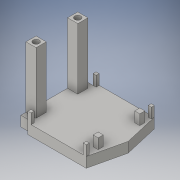
# Autodesk Inventor part: Maglev_Stand
Saved by Autodesk Inventor 2016 (Build 200138000, 138)
## iProperties
Created: 2018-01-06
Part Number: Maglev_Stand
Material: Generic
Document SubType Name: Modeling
Designer: Jorian Bruslind
Density: 1 g/cm^3
Appearance: Default
Author: Jorian Bruslind
Autodesk Inventor part; units mm, degrees
ref_plane "YZ Plane" through (0, 0, 0) normal (1, 0, 0) x (0, 1, 0)
ref_plane "XZ Plane" through (0, 0, 0) normal (0, 1, 0) x (-1, 0, 0)
ref_plane "XY Plane" through (0, 0, 0) normal (0, 0, 1) x (1, 0, 0)
sketch "Sketch1" plane through (0, 0, 0) normal (0, 1, 0) x (-1, 0, 0)
  line L0 (0, 0) -> (0, -85)
  line L1 (0, 0) -> (-60, 0)
  line L2 (-60, 0) -> (-60, -85)
  line L3 (-60, -85) -> (0, -85)
  line L4 (0, -42.5) -> (-76.2, -42.5)
  line L5 (-60, 0) -> (-66.35, 0)
  line L6 (-66.35, 0) -> (-66.35, -6.35)
  line L7 (-66.35, -6.35) -> (-60, -6.35)
  line L8 (-60, -6.35) -> (-60, 0)
  line L9 (0, 0) -> (6.35, 0)
  line L10 (6.35, 0) -> (6.35, -85)
  line L11 (6.35, -85) -> (0, -85)
  line L12 (-60, -85) -> (-66.35, -85)
  line L13 (-66.35, 0) -> (-76.2, -42.5)
  line L14 (-76.2, -42.5) -> (-66.35, -85)
  dimension "d0" = 85
  dimension "d1" = 60
  dimension "d2" = 76.2
  dimension "d3" = 6.35
  dimension "d4" = 6.35
  dimension "d5" = 6.35
  dimension "d6" = 6.35
  constraints: 30 end point, 4 perpendicular, 3 horizontal, 3 parallel, 2 vertical, 1 midpoint, 1 point on line
  measures "d0" distance of L0.start L0.end
  measures "d1" distance of L0.start L1.end
  measures "d2" distance of L4.start L4.end
  measures "d3" distance of L7.end L6.end
  measures "d4" distance of L6.end L5.end
  measures "d5" distance of L0.start L9.end
  measures "d6" distance of L2.end L12.end
extrude "Extrusion1" add sketch "Sketch1" along normal blind 12.7
sketch "Sketch2" plane through (0, 12.7, 0) normal (0, 1, 0) x (1, 0, 0)
  line L0 (-6.35, 0) -> (66.35, 0) projected
  line L1 (-6.35, 0) -> (-2.54, 0)
  line L2 (-2.54, 0) -> (-2.54, 3.81)
  line L3 (-2.54, 3.81) -> (-6.35, 3.81)
  line L4 (-6.35, 3.81) -> (-6.35, 0)
  line L5 (66.35, 85) -> (-6.35, 85) projected
  line L6 (-6.35, 85) -> (-2.54, 85)
  line L7 (-2.54, 85) -> (-2.54, 81.19)
  line L8 (-2.54, 81.19) -> (-6.35, 81.19)
  line L9 (-6.35, 81.19) -> (-6.35, 85)
  line L10 (66.35, 0) -> (62.54, 0)
  line L11 (62.54, 0) -> (62.54, 3.81)
  line L12 (62.54, 3.81) -> (66.35, 3.81)
  line L13 (66.35, 3.81) -> (66.35, 0)
  line L14 (66.35, 85) -> (62.54, 85)
  line L15 (62.54, 85) -> (62.54, 81.19)
  line L16 (62.54, 81.19) -> (66.35, 81.19)
  line L17 (66.35, 81.19) -> (66.35, 85)
  point P0 (0, 0)
  dimension "d9" = 3.81
  dimension "d10" = 3.81
  dimension "d11" = 3.81
  dimension "d12" = 3.81
  dimension "d13" = 3.81
  dimension "d14" = 3.81
  dimension "d15" = 3.81
  dimension "d16" = 3.81
  constraints: 32 end point, 8 parallel, 4 horizontal, 4 perpendicular
  measures "d9" distance of L3.end L2.end
  measures "d10" distance of L2.end L1.end
  measures "d11" distance of L7.end L8.end
  measures "d12" distance of L6.end L7.end
  measures "d13" distance of L11.end L12.end
  measures "d14" distance of L10.end L11.end
  measures "d15" distance of L16.end L15.end
  measures "d16" distance of L15.end L14.end
extrude "Extrusion2" add sketch "Sketch2" along normal blind 12.7
sketch "Sketch3" plane through (-6.35, 0, -85) normal (-1, 0, 0) x (0, 0, 1)
  line L0 (3.81, 12.7) -> (81.19, 12.7) projected
  line L1 (42.5, 0) -> (0, 0) projected
  line L2 (81.19, 12.7) -> (3.81, 12.7)
  line L3 (3.81, 12.7) -> (3.81, 0)
  line L4 (3.81, 0) -> (81.19, 0)
  line L5 (81.19, 0) -> (81.19, 12.7)
  point P0 (85, 0)
  constraints: 8 end point, 2 parallel, 1 horizontal, 1 perpendicular, 1 point on line
extrude "Extrusion3" add sketch "Sketch3" along normal blind 12.7
sketch "Sketch4" plane through (0, 12.7, 0) normal (0, 1, 0) x (1, 0, 0)
  line L0 (-19.05, 3.81) -> (-19.05, 10.16)
  line L1 (-19.05, 81.19) -> (-19.05, 3.81) projected
  line L2 (-19.05, 10.16) -> (-6.35, 10.16)
  line L3 (-6.35, 10.16) -> (-6.35, 22.86)
  line L4 (-6.35, 22.86) -> (-19.05, 22.86)
  line L5 (-19.05, 22.86) -> (-19.05, 10.16)
  line L6 (-6.35, 81.19) -> (-19.05, 81.19) projected
  line L7 (-19.05, 81.19) -> (-19.05, 74.84)
  line L8 (-19.05, 74.84) -> (-6.35, 74.84)
  line L9 (-6.35, 74.84) -> (-6.35, 62.14)
  line L10 (-6.35, 62.14) -> (-19.05, 62.14)
  line L11 (-19.05, 62.14) -> (-19.05, 74.84)
  dimension "d39" = 6.35
  dimension "d40" = 12.7
  dimension "d41" = 12.7
  dimension "d42" = 6.35
  dimension "d43" = 12.7
  dimension "d44" = 12.7
  constraints: 20 end point, 4 parallel, 2 horizontal, 2 perpendicular, 2 point on line
  measures "d39" distance of L0.start L0.end
  measures "d40" distance of L4.end L3.end
  measures "d41" distance of L3.end L2.end
  measures "d42" distance of L1.start L7.end
  measures "d43" distance of L9.end L10.end
  measures "d44" distance of L8.end L9.end
extrude "Extrusion4" add sketch "Sketch4" along normal blind 76.2
sketch "Sketch5" plane through (0, 88.9, 0) normal (0, 1, 0) x (1, 0, 0)
  line L0 (-2.54, 3.81) -> (-6.35, 3.81) projected
  line L1 (-19.05, 74.84) -> (-19.05, 81.19) projected
  line L2 (-19.05, 74.84) -> (-19.05, 68.49)
  line L3 (-19.05, 81.19) -> (-19.05, 3.81) projected
  line L4 (-19.05, 68.49) -> (-12.7, 68.49)
  circle A0 centre (-12.7, 68.49) radius 3.81
  line L5 (-19.05, 22.86) -> (-19.05, 62.14) projected
  line L6 (-19.05, 22.86) -> (-19.05, 16.51)
  line L7 (-19.05, 16.51) -> (-12.7, 16.51)
  circle A1 centre (-12.7, 16.51) radius 3.81
  point P0 (0, 0)
  point P1 (-6.35, 68.49)
  dimension "d45" = 6.35
  dimension "d46" = 6.35
  dimension "d47" = 7.62
  dimension "d48" = 6.35
  dimension "d49" = 6.35
  dimension "d50" = 7.62
  constraints: 8 end point, 2 centre point, 2 coincident, 2 point on line, 1 horizontal, 1 perpendicular
  measures "d45" distance of L1.start L2.end
  measures "d46" distance of L2.end L4.end
  measures "d47" diameter of A0
  measures "d48" distance of L5.start L6.end
  measures "d49" distance of L6.end L7.end
  measures "d50" diameter of A1
extrude "Extrusion5" cut sketch "Sketch5" against normal blind 25.4
sketch "Sketch6" plane through (0, 12.7, 0) normal (0, 1, 0) x (1, 0, 0)
  line L0 (62.54, 3.81) -> (66.35, 3.81) projected
  line L1 (66.35, 3.81) -> (66.35, 14.9225)
  line L2 (66.35, 81.19) -> (62.54, 81.19) projected
  line L3 (66.35, 81.19) -> (66.35, 73.2398)
  line L4 (66.35, 14.9225) -> (60, 14.9225)
  line L5 (60, 14.9225) -> (60, 21.2725)
  line L6 (60, 21.2725) -> (66.35, 21.2725)
  line L7 (66.35, 21.2725) -> (66.35, 14.9225)
  line L8 (66.35, 73.2398) -> (60, 73.2398)
  line L9 (60, 73.2398) -> (60, 66.8898)
  line L10 (60, 66.8898) -> (66.35, 66.8898)
  line L11 (66.35, 66.8898) -> (66.35, 73.2398)
  point P0 (0, 0)
  dimension "d31" = 11.1125
  dimension "d32" = 7.9502
  dimension "d33" = 6.35
  dimension "d34" = 6.35
  dimension "d35" = 6.35
  dimension "d36" = 6.35
  constraints: 20 end point, 4 parallel, 2 horizontal, 2 perpendicular, 2 vertical
  measures "d31" distance of L0.end L1.end
  measures "d32" distance of L2.start L3.end
  measures "d33" distance of L5.end L6.end
  measures "d34" distance of L4.end L5.end
  measures "d35" distance of L10.end L9.end
  measures "d36" distance of L9.end L8.end
extrude "Extrusion6" add sketch "Sketch6" along normal blind 12.7
body "Solid1"
